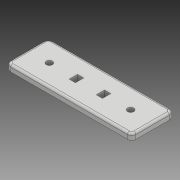
# Autodesk Inventor part: tapa_soporte_bateria
Saved by Autodesk Inventor 2018 (Build 220112000, 112)
## iProperties
Created: 2019-01-15
Part Number: tapa_soporte_bateria
Material: Genérico
Document SubType Name: Modeling
Designer: becar
Density: 1 g/cm^3
Appearance: Valor por defecto
Author: becar
Autodesk Inventor part; units mm, degrees
ref_plane "YZ Plane" through (0, 0, 0) normal (1, 0, 0) x (0, 1, 0)
ref_plane "XZ Plane" through (0, 0, 0) normal (0, 1, 0) x (-1, 0, 0)
ref_plane "XY Plane" through (0, 0, 0) normal (0, 0, 1) x (1, 0, 0)
sketch "Boceto1" plane through (0, 0, 0) normal (0, 0, 1) x (1, 0, 0)
  line L0 (0, 0) -> (60, 0)
  line L1 (60, 0) -> (60, 20)
  line L2 (60, 20) -> (0, 20)
  line L3 (0, 20) -> (0, 0)
  line L4 (30, 20) -> (10.5, 20)
  line L5 (30, 20) -> (49.5, 20)
  line L6 (49.5, 20) -> (49.5, 10)
  circle A0 centre (10.5, 10) radius 1.5
  circle A1 centre (49.5, 10) radius 1.5
  line L7 (30, 20) -> (35, 20)
  line L8 (35, 20) -> (35, 10)
  line L9 (38, 10) -> (38, 12)
  line L10 (38, 10) -> (38, 8)
  line L11 (38, 8) -> (35, 8)
  line L12 (35, 8) -> (35, 10)
  line L13 (38, 12) -> (35, 12)
  line L14 (30, 20) -> (25, 20)
  line L15 (25, 20) -> (25, 12)
  line L16 (25, 12) -> (25, 8)
  line L17 (25, 8) -> (22, 8)
  line L18 (22, 8) -> (22, 12)
  line L19 (22, 12) -> (25, 12)
  dimension "d0" = 60
  dimension "d1" = 20
  dimension "d2" = 19.5
  dimension "d3" = 19.5
  dimension "d4" = 10
  dimension "d5" = 3
  dimension "d6" = 3
  dimension "d7" = 5
  dimension "d8" = 3
  dimension "d9" = 2
  dimension "d10" = 2
  dimension "d11" = 5
  dimension "d12" = 3
  constraints: 40 end point, 12 perpendicular, 6 point on line, 2 centre point, 2 vertical, 1 coincident, 1 horizontal, 1 midpoint
  measures "d0" distance of L0.start L0.end
  measures "d1" distance of L0.end L1.end
  measures "d2" distance of L4.start L4.end
  measures "d3" distance of L4.start L5.end
  measures "d4" distance of L5.end L6.end
  measures "d5" diameter of A0
  measures "d6" diameter of A1
  measures "d7" distance of L4.start L7.end
  measures "d8" distance of L8.end L9.start
  measures "d9" distance of L9.start L9.end
  measures "d10" distance of L9.start L10.end
  measures "d11" distance of L4.start L14.end
  measures "d12" distance of L16.end L17.end
extrude "Extrusión1" add sketch "Boceto1" along normal blind 3
fillet "Empalme1" radius 2 4 edges at (60, 20, 1.5) (60, 0, 1.5) (0, 20, 1.5) (0, 0, 1.5)
fillet "Empalme2" radius 1 8 edges at (0.5858, 19.4142, 3) (0, 10, 3) (0.5858, 0.5858, 3) (30, 0, 3) (59.4142, 0.5858, 3) (60, 10, 3) (59.4142, 19.4142, 3) (42.25, 20, 3)
